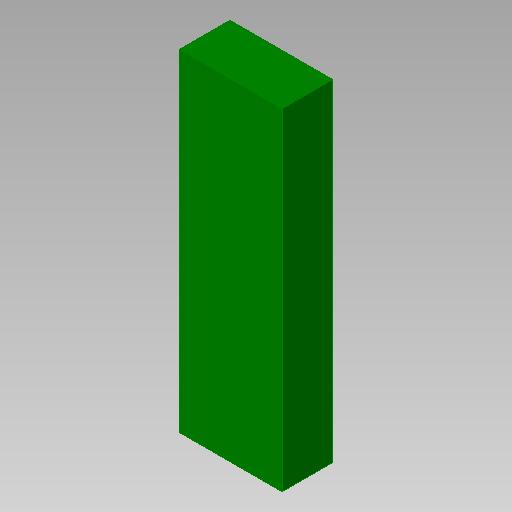
# Autodesk Inventor part: 32_768KHZ
Saved by Autodesk Inventor 2020.1 (Build 241239000, 239)
## iProperties
Created: 2015-11-24
Part Number: 32_768KHZ
Material: Generic
Document SubType Name: Modeling
Designer: PhillipD
Density: 1 g/cm^3
Appearance: MS3V-T1R, 32_768KHZ
Author: PhillipD
Autodesk Inventor part; units mm, degrees
ref_plane "YZ Plane" through (0, 0, 0) normal (1, 0, 0) x (0, 1, 0)
ref_plane "XZ Plane" through (0, 0, 0) normal (0, 1, 0) x (-1, 0, 0)
ref_plane "XY Plane" through (0, 0, 0) normal (0, 0, 1) x (1, 0, 0)
sketch "MS3V-T1R, 32_768KHZ_91" plane through (0, 0, 0) normal (0, 0, 1) x (1, 0, 0)
  line L0 (-1.016, 2.887) -> (1.016, 2.887)
  line L1 (1.016, 2.887) -> (1.016, -3.6752)
  line L2 (1.016, -3.6752) -> (-1.016, -3.6752)
  line L3 (-1.016, -3.6752) -> (-1.016, 2.887)
  constraints: 8 end point
extrude "Extrusion1" add sketch "MS3V-T1R, 32_768KHZ_91" along normal blind 1
body "Solid1"
